Axle Hub_v1 (Autodesk Fusion 360 design; units mm, degrees)
Autodesk Fusion 360 part; units mm, degrees
sketch "Sketch1" plane through (0, 0, 0) normal (0, 0, 1) x (1, 0, 0)
  circle A0 centre (0, 0) radius 28 construction
  circle A1 centre (0, -28) radius 2
  circle A2 centre (16.458, -22.6525) radius 2
  circle A3 centre (26.6296, -8.6525) radius 2
  circle A4 centre (26.6296, 8.6525) radius 2
  circle A5 centre (16.458, 22.6525) radius 2
  circle A6 centre (0, 28) radius 2
  circle A7 centre (-16.458, 22.6525) radius 2
  circle A8 centre (-26.6296, 8.6525) radius 2
  circle A9 centre (-26.6296, -8.6525) radius 2
  circle A10 centre (-16.458, -22.6525) radius 2
  circle A11 centre (0, 0) radius 33
  circle A12 centre (0, 0) radius 23
  dimension "d1" = 56
  dimension "d2" = 4
  dimension "d4" = 360
  dimension "d5" = 66
  dimension "d6" = 46
  constraint coincident A0.centre A11.centre
  constraint coincident A0 A1.centre
  constraint concentric A0 A11
  constraint concentric A11 A12
  measures "d1" diameter of A0
  measures "d2" diameter of A1
  measures "d5" diameter of A11
  measures "d6" diameter of A12
extrude "Extrude1" add sketch "Sketch1" along normal blind 7
equation "d5 = d1 + 10 mm"
equation "d6 = d1 - 10 mm"
